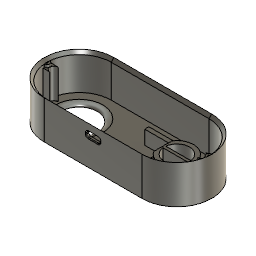
controller_main_part (Autodesk Fusion 360 design; units mm, degrees)
part number: 2025-12-25-17-05-01-501
Autodesk Fusion 360 part; units mm, degrees
sketch "Skizze1" plane through (0, 0, 0) normal (0, 0, 1) x (1, 0, 0)
  line L0 (25, 25) -> (95, 25)
  line L1 (95, 25) -> (95, 75)
  line L2 (95, 75) -> (25, 75)
  line L3 (25, 75) -> (25, 25)
  circle A0 centre (25, 50) radius 25
  circle A1 centre (95, 50) radius 25
  dimension "d1" = 70
  dimension "d2" = 50
  constraint horizontal L0
  constraint vertical L1
  constraint horizontal L2
  constraint vertical L3
  constraint midpoint L3 A0.centre
  constraint coincident L0.start A0
  constraint midpoint L1 A1.centre
  constraint coincident L0.end A1
  measures "d1" distance of L0.start L0.end
  measures "d2" distance of L0.start L2.end
extrude "Extrusion1" add sketch "Skizze1" along normal blind 25.5
extrude "Extrusion2" add 1 faces at (71.6667, 41.6667, 25.5) along direction (0, 0, 1) blind 1
extrude "Extrusion3" add 1 faces at (71.6667, 41.6667, 26.5) along direction (0, 0, 1) blind 1
extrude "Extrusion4" cut 1 faces at (71.6667, 41.6667, 27.5) along direction (0, 0, -1) blind 2 draft -45
extrude "Extrusion5" cut 1 faces at (71.6667, 42.3333, 25.5) along direction (0, 0, -1) blind 23.5
sketch "Skizze2" plane through (0, 0, 2) normal (0, 0, 1) x (-1, 0, 0)
  line L0 (-95, -73) -> (-25, -73)
  arc A0 (-25, -73) -> (-25, -27) centre (-25, -50) ccw
  line L1 (-25, -27) -> (-95, -27)
  arc A1 (-95, -27) -> (-95, -73) centre (-95, -50) ccw
  line L2 (-25, -73) -> (-25, -27)
  circle A2 centre (-25, -50) radius 13
  line L3 (-95, -73) -> (-95, -27)
  circle A3 centre (-95, -50) radius 9
  line L4 (-95, -50) -> (-95, -51)
  line L5 (-95, -51) -> (-86.0557, -51)
  line L6 (-95, -51) -> (-103.9443, -51)
  line L7 (-95, -50) -> (-95, -49)
  line L8 (-95, -49) -> (-86.0557, -49)
  line L9 (-95, -49) -> (-103.9443, -49)
  dimension "d13" = 26
  dimension "d14" = 18
  constraint coincident L0.end A0.start
  constraint coincident A0.end L1.start
  constraint concentric A0 A2
  constraint coincident L0.start A1.end
  constraint coincident L1.end A1.start
  constraint concentric A1 A3
  constraint coincident A1.centre A3.centre
  constraint parallel L3 L4
  constraint coincident A3 L5.end
  constraint perpendicular L3 L5
  constraint coincident A3 L6.end
  constraint perpendicular L3 L6
  constraint parallel L3 L7
  constraint coincident A3 L8.end
  constraint perpendicular L3 L8
  constraint coincident A3 L9.end
  constraint perpendicular L7 L9
  measures "d13" diameter of A2
  measures "d14" diameter of A3
extrude "Extrusion6" cut sketch "Skizze2" against normal blind 2 contours L3 A3 L6 | L3 A3 L5 | L3 A3 L8 | L3 A3 L9
extrude "Extrusion7" cut sketch "Skizze2" against normal blind 2 contours L2 A2 | L2 A2
fillet "Abrundung1" offset 4 second offset 2 tangency weight 0.5 1 edges at (37.1203, 45.299, 2) measured on face at (72.9431, 37.9708, 2)
sketch "Skizze4" plane through (0, 25, 0) normal (0, -1, 0) x (1, 0, 0)
  line L0 (25, 0) -> (95, 0)
  line L1 (95, 0) -> (95, 27.5)
  line L2 (95, 27.5) -> (25, 27.5)
  line L3 (25, 27.5) -> (25, 0)
  line L4 (65, 20.8) -> (65, 19.8)
  line L5 (63.5, 18.3) -> (56.5, 18.3)
  line L6 (55, 19.8) -> (55, 20.8)
  arc A0 (55, 19.8) -> (56.5, 18.3) centre (56.5, 19.8) ccw
  arc A1 (56.5, 22.3) -> (55, 20.8) centre (56.5, 20.8) ccw
  arc A2 (65, 20.8) -> (63.5, 22.3) centre (63.5, 20.8) ccw
  arc A3 (63.5, 18.3) -> (65, 19.8) centre (63.5, 19.8) ccw
  line L7 (56.5, 22.3) -> (63.5, 22.3)
  dimension "d30" = 1.5
  dimension "d31" = 1.5
  dimension "d32" = 1.5
  dimension "d33" = 1.5
  constraint vertical L4
  constraint horizontal L5
  constraint vertical L6
  constraint tangent L6 A0
  constraint tangent L5 A0
  constraint tangent L6 A1
  constraint tangent L4 A2
  constraint tangent L5 A3
  constraint tangent L4 A3
  constraint tangent A2 L7
  measures "d30" radius of A0
  measures "d31" radius of A1
  measures "d32" radius of A2
  measures "d33" radius of A3
extrude "Extrusion8" cut sketch "Skizze4" against normal blind 2 contours L4 L5 L6 A0 A1 A2 A3 L7
fillet "Abrundung2" radius 0.5 curvature continuous 8 edges at (60, 25, 22.3) (64.5607, 25, 21.8607) (65, 25, 20.3) (64.5607, 25, 18.7393) (60, 25, 18.3) (55.4393, 25, 18.7393) (55, 25, 20.3) (55.4393, 25, 21.8607)
sketch "Skizze5" plane through (0, 0, 2) normal (0, 0, 1) x (-1, 0, 0)
  line L0 (-95, -73) -> (-25, -73)
  arc A0 (-25, -73) -> (-25, -27) centre (-25, -50) ccw
  line L1 (-25, -27) -> (-95, -27)
  arc A1 (-95, -27) -> (-95, -73) centre (-95, -50) ccw
  arc A2 (-103.9443, -51) -> (-86.0557, -51) centre (-95, -50) ccw
  line L2 (-103.9443, -51) -> (-86.0557, -51)
  line L3 (-86.0557, -49) -> (-103.9443, -49)
  arc A3 (-86.0557, -49) -> (-103.9443, -49) centre (-95, -50) ccw
  spline S0 degree 3 poles (-42, -50) (-42, -51.4301) (-41.8186, -52.8601) (-40.6834, -57.2623) (-39.0565, -60.056) (-34.5929, -64.3715) (-31.7721, -65.8966) (-25.7294, -67.2655) (-22.5151, -67.1013) (-16.6782, -65.1356) (-14.0554, -63.3624) (-10.0729, -58.6979) (-8.7283, -55.8053) (-7.7412, -49.8264) (-8.0478, -46.7568) (-10.1796, -41.1392) (-12.0247, -38.6071) (-16.6042, -34.9484) (-19.2691, -33.7459) (-24.9417, -32.7505) (-27.9513, -33.0048) (-33.0998, -34.8391) (-35.298, -36.2373) (-38.9985, -39.9779) (-40.4369, -42.3776) (-41.7431, -46.6002) (-42, -48.3) (-42, -50) knots -3.141593 -3.141593 -3.141593 -3.141593 -2.889223 -2.889223 -2.339318 -2.339318 -1.793572 -1.793572 -1.245952 -1.245952 -0.70668 -0.70668 -0.163612 -0.163612 0.362702 0.362702 0.896709 0.896709 1.397099 1.397099 1.913058 1.913058 2.361593 2.361593 2.841593 2.841593 3.141593 3.141593 3.141593 3.141593
  circle A4 centre (-2, -50) radius 2
  circle A5 centre (-118, -50) radius 2
extrude "Extrusion9" add sketch "Skizze5" along normal blind 22.5 contours A0 A4 picked at (-2.6713, -50.0484)
extrude "Extrusion10" add 1 faces at (2.6713, 50.0484, 24.5) along direction (0, 0, 1) blind 1
extrude "Extrusion11" add sketch "Skizze5" along normal blind 23.5 contours A1 A5 picked at (-117.3269, -50)
hole "Bohrung1" at (118, 50, 25.5) direction (0, 0, -1) diameter 1.5 depth 6 tip angle 118
hole "Bohrung2" at (2, 50, 25.5) direction (0, 0, -1) diameter 1.5 depth 6 tip angle 118
sketch "Skizze7" plane through (0, 0, 2) normal (0, 0, 1) x (-1, 0, 0)
  spline S0 degree 3 poles (-42, -50) (-42, -51.4301) (-41.8186, -52.8601) (-40.6834, -57.2623) (-39.0565, -60.056) (-34.5929, -64.3715) (-31.7721, -65.8966) (-25.7294, -67.2655) (-22.5151, -67.1013) (-16.6782, -65.1356) (-14.0554, -63.3624) (-10.0729, -58.6979) (-8.7283, -55.8053) (-7.7412, -49.8264) (-8.0478, -46.7568) (-10.1796, -41.1392) (-12.0247, -38.6071) (-16.6042, -34.9484) (-19.2691, -33.7459) (-24.9417, -32.7505) (-27.9513, -33.0048) (-33.0998, -34.8391) (-35.298, -36.2373) (-38.9985, -39.9779) (-40.4369, -42.3776) (-41.7431, -46.6002) (-42, -48.3) (-42, -50) knots -3.141593 -3.141593 -3.141593 -3.141593 -2.889223 -2.889223 -2.339318 -2.339318 -1.793572 -1.793572 -1.245952 -1.245952 -0.70668 -0.70668 -0.163612 -0.163612 0.362702 0.362702 0.896709 0.896709 1.397099 1.397099 1.913058 1.913058 2.361593 2.361593 2.841593 2.841593 3.141593 3.141593 3.141593 3.141593
  line L0 (-86.0557, -49) -> (-103.9443, -49)
  arc A0 (-86.0557, -49) -> (-103.9443, -49) centre (-95, -50) ccw
  arc A1 (-103.9443, -51) -> (-86.0557, -51) centre (-95, -50) ccw
  line L1 (-103.9443, -51) -> (-86.0557, -51)
  arc A2 (-117.913, -51.9981) -> (-117.913, -48.0019) centre (-118, -50) ccw
  arc A3 (-117.913, -51.9981) -> (-95, -73) centre (-95, -50) ccw
  line L2 (-95, -73) -> (-25, -73)
  arc A4 (-25, -73) -> (-2.087, -51.9981) centre (-25, -50) ccw
  arc A5 (-2.087, -48.0019) -> (-2.087, -51.9981) centre (-2, -50) ccw
  arc A6 (-2.087, -48.0019) -> (-25, -27) centre (-25, -50) ccw
  line L3 (-25, -27) -> (-95, -27)
  arc A7 (-95, -27) -> (-117.913, -48.0019) centre (-95, -50) ccw
  circle A8 centre (-113, -50) radius 3
  line L4 (-113, -53) -> (-117.8035, -53)
  line L5 (-113, -47) -> (-117.8035, -47)
  circle A9 centre (-7, -50) radius 3
  line L6 (-7, -47) -> (-2.1965, -47)
  line L7 (-7, -53) -> (-2.1965, -53)
  line L8 (-60, -27) -> (-45, -27)
  line L9 (-45, -27) -> (-85, -27)
  line L10 (-85, -27) -> (-85, -57)
  line L11 (-85, -57) -> (-45, -57)
  line L12 (-45, -57) -> (-45, -27)
  line L13 (-65, -57) -> (-65, -62)
  line L14 (-65, -62) -> (-85, -62)
  line L15 (-85, -62) -> (-85, -57)
  line L16 (-85, -57) -> (-65, -57)
  line L17 (-65, -57) -> (-65, -62)
  line L18 (-85, -27) -> (-90, -27)
  line L19 (-90, -27) -> (-90, -37)
  line L20 (-90, -37) -> (-85, -37)
  line L21 (-85, -37) -> (-85, -27)
  line L22 (-45, -27) -> (-40, -27)
  line L23 (-40, -27) -> (-40, -32)
  line L24 (-40, -32) -> (-45, -32)
  line L25 (-45, -32) -> (-45, -27)
  circle A10 centre (-95, -50) radius 12
  line L26 (-90, -37) -> (-90, -39.0913)
  line L27 (-85, -62) -> (-95, -62)
  dimension "d60" = 15
  dimension "d61" = 40
  dimension "d62" = 30
  dimension "d63" = 5
  dimension "d64" = 5
  dimension "d65" = 10
  dimension "d66" = 5
  dimension "d67" = 5
  constraint coincident A8 L4.start
  constraint coincident A3 L4.end
  constraint coincident A8 L5.start
  constraint coincident A7 L5.end
  constraint parallel L4 L5
  constraint coincident A9 L6.start
  constraint coincident A6 L6.end
  constraint coincident A9 L7.start
  constraint coincident A4 L7.end
  constraint parallel L6 L7
  constraint midpoint L3 L8.start
  constraint parallel L3 L8
  constraint horizontal L9
  constraint vertical L10
  constraint horizontal L11
  constraint vertical L12
  constraint midpoint L11 L13.start
  constraint perpendicular L11 L13
  constraint horizontal L14
  constraint vertical L15
  constraint horizontal L16
  constraint vertical L17
  constraint horizontal L18
  constraint vertical L19
  constraint horizontal L20
  constraint vertical L21
  constraint horizontal L22
  constraint vertical L23
  constraint horizontal L24
  constraint vertical L25
  constraint concentric A0 A10
  constraint coincident A10 L26.end
  constraint perpendicular L20 L26
  constraint coincident A10 L27.end
  constraint tangent A10 L27
  constraint perpendicular L15 L27
  measures "d60" distance of L8.start L8.end
  measures "d61" distance of L8.end L9.end
  measures "d62" distance of L8.end L11.end
  measures "d63" distance of L13.start L13.end
  measures "d64" distance of L9.end L18.end
  measures "d65" distance of L9.end L20.end
  measures "d66" distance of L8.end L22.end
  measures "d67" distance of L8.end L24.end
extrude "Extrusion12" add sketch "Skizze7" along normal blind 21.5 contours A4 A5 A9 L7 | A5 A6 A9 L6 | A2 A3 A8 L4 | A2 A7 A8 L5
extrude "Extrusion13" add sketch "Skizze7" along normal blind 10 contours L3 L12 L22 L23 L24 L25
extrude "Extrusion14" add sketch "Skizze7" along normal blind 10 contours L11 L13 L14 L15 L16 L17
extrude "Extrusion15" add sketch "Skizze7" along normal blind 10 contours L3 L10 L18 L19 L20 L21
extrude "Extrusion16" add sketch "Skizze7" along normal blind 13 contours L10 A10 picked at (-92.0186, -49.6667)
extrude "Extrusion17" add sketch "Skizze7" along normal blind 10 contours L10 L20 A10 L26 | L10 L15 A10 L27
extrude "Extrusion18" cut 1 faces at (75, 62, 5.3333) along direction (0, -1, 0) blind 2
extrude "Extrusion19" add 1 faces at (95, 60.6667, 5.3333) along direction (-1, 0, 0) blind 6
extrude "Extrusion20" cut 1 faces at (89.4693, 61.1596, 12) along direction (0, 0, -1) blind 10
